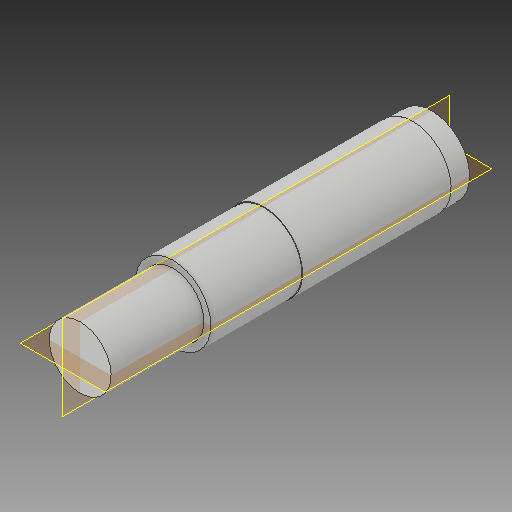
# Autodesk Inventor part: Вал тихоходный
Saved by Autodesk Inventor 2018 (Build 220112000, 112)
## iProperties
Created: 2018-03-24
Part Number: Вал тихоходный
Material: Типовые
Document SubType Name: Modeling
Designer: kriku
Density: 1 g/cm^3
Appearance: По умолчанию
Author: kriku
Autodesk Inventor part; units mm, degrees
ref_plane "XY Plane" through (0, 0, 0) normal (0, 0, 1) x (1, 0, 0)
sketch "Эскиз1" plane through (0, 0, 0) normal (1, 0, 0) x (0, 1, 0)
  line L0 (22.5, 95.625) -> (22.5, 28.125)
  line L1 (22.5, 28.125) -> (27.5, 28.125)
  line L2 (27.5, 28.125) -> (27.5, -38.065)
  line L3 (27.5, -38.065) -> (28, -38.065)
  line L4 (28, -38.065) -> (28, -146.065)
  line L5 (28, -146.065) -> (27.5, -146.065)
  line L6 (27.5, -146.065) -> (27.5, -160.0374)
  line L7 (27.5, -160.0374) -> (0, -160.0374)
  line L8 (0, -160.0374) -> (0, 95.625)
  line L9 (0, 95.625) -> (22.5, 95.625)
  point P0 (0, 0)
  dimension "d0" = 45
  dimension "d1" = 55
  dimension "d2" = 56
  dimension "d3" = 67.5
  dimension "d4" = 66.19
  dimension "d5" = 108
  constraints: 20 end point, 8 perpendicular, 2 point on line, 1 vertical
  measures "d0" diameter of L0 L8
  measures "d1" diameter of L2 L8
  measures "d2" diameter of L4 L8
  measures "d3" distance of L0.start L0.end
  measures "d4" distance of L1.end L2.end
  measures "d5" distance of L3.end L4.end
revolve "Вращение1" add sketch "Эскиз1" angle 360 about axis through (0, 0, -160.0374) along (0, 0, 1)
